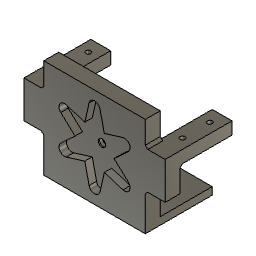
Middle_Servo_Mount (Autodesk Fusion 360 design; units mm, degrees)
Autodesk Fusion 360 part; units mm, degrees
note: some values were not read from the file. Set by a fixed rule: which sketch regions a step uses.
sketch "Sketch1" plane through (0, 0, 0) normal (0, 0, 1) x (1, 0, 0)
  line L0 (41, 21) -> (20.5, 21)
  line L1 (20.5, 21) -> (0, 21)
  line L2 (41, 0) -> (41, 21)
  line L3 (0, 21) -> (0, 0)
  line L4 (0, 0) -> (41, 0)
  dimension "d1" = 21
  dimension "d2" = 41
  constraint horizontal L4
  constraint vertical L2
  constraint horizontal L0
  constraint vertical L3
  constraint coincident L3.end L4.start
  constraint collinear L0 L1
  measures "d1" distance of L3.end L1.end
  measures "d2" distance of L3.end L2.start
extrude "Extrude1" add sketch "Sketch1" along normal blind 3
sketch "Sketch7" plane through (0, 0, 0) normal (0, 0, -1) x (1, 0, 0)
  line L0 (0, 0) -> (0, -21)
  line L1 (0, -21) -> (20.5, -21)
  line L2 (20.5, -21) -> (41, -21)
  line L3 (41, -21) -> (41, 0)
  line L4 (41, 0) -> (0, 0)
  line L5 (0, 0) -> (41, 0)
  line L6 (41, 0) -> (41, 6)
  line L7 (41, 6) -> (0, 6)
  line L8 (0, 6) -> (0, 0)
  dimension "d23" = 6
  constraint horizontal L5
  constraint vertical L6
  constraint horizontal L7
  constraint vertical L8
  measures "d23" distance of L3.end L6.end
extrude "Extrude6" add sketch "Sketch7" against normal blind 40 contours L4 L5 L6 L7 L8
sketch "Sketch8" plane through (0, -6, 0) normal (0, -1, 0) x (1, 0, 0)
  line L0 (0, 0) -> (41, 0)
  line L1 (41, 0) -> (41, 40)
  line L2 (41, 40) -> (0, 40)
  line L3 (0, 40) -> (0, 0)
  line L4 (41, 15) -> (49, 15)
  line L5 (49, 15) -> (49, 30)
  line L6 (49, 30) -> (41, 30)
  line L7 (41, 30) -> (41, 15)
  line L8 (20.5, 40) -> (20.5, 3)
  line L9 (0, 15) -> (-8, 15)
  line L10 (-8, 15) -> (-8, 30)
  line L11 (-8, 30) -> (0, 30)
  line L12 (0, 3) -> (41, 3)
  line L13 (0, 3) -> (41, 3)
  line L14 (0, 3) -> (41, 3)
  line L15 (0, 3) -> (41, 3)
  dimension "d24" = 15
  dimension "d25" = 27
  dimension "d28" = 8
  constraint horizontal L4
  constraint vertical L5
  constraint horizontal L6
  constraint vertical L7
  constraint coincident L1 L4.start
  constraint midpoint L2 L8.start
  constraint symmetric L4.start L8 L9.start
  constraint symmetric L4.end L8 L9.end
  constraint symmetric L5.end L8 L10.end
  constraint symmetric L6.end L8 L11.end
  measures "d24" distance of L4.end L5.end
  measures "d25" distance of L6 L12.end
  measures "d28" distance of L4.start L4.end
extrude "Extrude7" add sketch "Sketch8" against normal up to surface (6 mm away) contours L3 L9 L10 L11 | L1 L4 L5 L6 L7
sketch "Sketch9" plane through (0, 0, 0) normal (0, 1, 0) x (-1, 0, 0)
  line L0 (-41, 3) -> (0, 3)
  line L1 (0, 3) -> (0, 15)
  line L2 (0, 15) -> (8, 15)
  line L3 (8, 15) -> (8, 30)
  line L4 (8, 30) -> (0, 30)
  line L5 (0, 30) -> (0, 40)
  line L6 (0, 40) -> (-41, 40)
  line L7 (-41, 40) -> (-41, 30)
  line L8 (-41, 30) -> (-49, 30)
  line L9 (-49, 30) -> (-49, 15)
  line L10 (-49, 15) -> (-41, 15)
  line L11 (-41, 15) -> (-41, 3)
  line L12 (-49, 30) -> (-41, 30)
  line L13 (-41, 30) -> (-41, 25)
  line L14 (-41, 25) -> (-49, 25)
  line L15 (-49, 25) -> (-49, 30)
  line L16 (8, 30) -> (0, 30)
  line L17 (0, 30) -> (0, 25)
  line L18 (0, 25) -> (8, 25)
  line L19 (8, 25) -> (8, 30)
  dimension "d29" = 5
  dimension "d54" = 5
  constraint horizontal L12
  constraint vertical L13
  constraint horizontal L14
  constraint vertical L15
  constraint coincident L8.end L9.start
  constraint horizontal L16
  constraint vertical L17
  constraint horizontal L18
  constraint vertical L19
  constraint coincident L3.end L4.start
  measures "d29" distance of L7.end L13.end
  measures "d54" distance of L4.end L17.end
extrude "Extrude8" add sketch "Sketch9" along normal up to surface (21 mm away) contours L8 L9 L12 L13 L14 L15 | L3 L4 L16 L17 L18 L19
sketch "Sketch10" plane through (0, 0, 30) normal (0, 0, 1) x (-1, 0, 0)
  line L0 (8, -21) -> (8, 6)
  line L1 (8, 6) -> (0, 6)
  line L2 (0, 6) -> (0, 0)
  line L3 (0, 0) -> (0, -21)
  line L4 (0, -21) -> (8, -21)
  circle A0 centre (4, -16) radius 1
  circle A1 centre (4, -5) radius 1
  circle A2 centre (-45, -16) radius 1
  circle A3 centre (-45, -5) radius 1
  line L5 (-41, 0) -> (-41, -21)
  line L6 (0, 0) -> (-41, 0)
  dimension "d32" = 2
  dimension "d33" = 5
  dimension "d34" = 4
  dimension "d36" = 4
  dimension "d39" = 5
  constraint equal A0 A1
  constraint equal A0 A2
  constraint equal A0 A3
  constraint vertical A0.centre A1.centre
  constraint horizontal A0.centre A2.centre
  constraint horizontal A1.centre A3.centre
  constraint vertical A2.centre A3.centre
  measures "d32" diameter of A0
  measures "d33" distance of L4 A0.centre
  measures "d34" distance of L3 A0.centre
  measures "d36" distance of A2.centre L5
  measures "d39" distance of A1.centre L6
extrude "Extrude9" cut sketch "Sketch10" against normal blind 5 contours A0 | A1 | A2 | A3
chamfer "Chamfer1" distance 1 angle 45 2 edges at (-4, 0, 25) (45, 0, 25)
chamfer "Chamfer2" distance 1 angle 45 4 edges at (0, -3, 15) (41, -3, 15) (41, -3, 30) (0, -3, 30)
sketch "Sketch14" plane through (0, -6, 0) normal (0, -1, 0) x (1, 0, 0)
  line L0 (0, 0) -> (41, 0)
  line L1 (41, 0) -> (41, 14)
  line L2 (41, 14) -> (42, 15)
  line L3 (42, 15) -> (49, 15)
  line L4 (49, 15) -> (49, 30)
  line L5 (49, 30) -> (42, 30)
  line L6 (42, 30) -> (41, 31)
  line L7 (41, 31) -> (41, 40)
  line L8 (41, 40) -> (0, 40)
  line L9 (0, 40) -> (0, 31)
  line L10 (0, 31) -> (-1, 30)
  line L11 (-1, 30) -> (-8, 30)
  line L12 (-8, 30) -> (-8, 15)
  line L13 (-8, 15) -> (-1, 15)
  line L14 (-1, 15) -> (0, 14)
  line L15 (0, 14) -> (0, 0)
  line L16 (6.8481, 25.348) -> (12.6318, 20)
  line L17 (12.6318, 20) -> (6.8481, 14.652)
  arc A0 (6.8481, 14.652) -> (9.0425, 10.8511) centre (8.3756, 13) ccw
  line L18 (9.0425, 10.8511) -> (16.5659, 13.1859)
  line L19 (16.5659, 13.1859) -> (18.3056, 5.5031)
  arc A1 (18.3056, 5.5031) -> (22.6944, 5.5031) centre (20.5, 6) ccw
  line L20 (22.6944, 5.5031) -> (24.4341, 13.1859)
  line L21 (24.4341, 13.1859) -> (31.9575, 10.8511)
  arc A2 (31.9575, 10.8511) -> (34.1519, 14.652) centre (32.6244, 13) ccw
  line L22 (34.1519, 14.652) -> (28.3682, 20)
  line L23 (28.3682, 20) -> (34.1519, 25.348)
  arc A3 (34.1519, 25.348) -> (31.9575, 29.1489) centre (32.6244, 27) ccw
  line L24 (31.9575, 29.1489) -> (24.4341, 26.8141)
  line L25 (24.4341, 26.8141) -> (22.6944, 34.4969)
  arc A4 (22.6944, 34.4969) -> (18.3056, 34.4969) centre (20.5, 34) ccw
  line L26 (18.3056, 34.4969) -> (16.5659, 26.8141)
  line L27 (16.5659, 26.8141) -> (9.0425, 29.1489)
  arc A5 (9.0425, 29.1489) -> (6.8481, 25.348) centre (8.3756, 27) ccw
  point P0 (20.5, 20)
  dimension "d48" = 40
  dimension "d49" = 41
  measures "d48" distance of L0.start L8.end
  measures "d49" distance of L0.start L0.end
extrude "Extrude11" cut sketch "Sketch14" against normal blind 3 contours L16 L17 A0 L18 L19 A1 L20 L21 A2 L22 L23 A3 L24 L25 A4 L26 L27 A5
sketch "Sketch15" plane through (0, 0, 0) normal (0, 1, 0) x (-1, 0, 0)
  line L0 (-41, 24) -> (-49, 24)
  line L1 (-49, 24) -> (-49, 15)
  line L2 (-49, 15) -> (-42, 15)
  line L3 (-42, 15) -> (-41, 14)
  line L4 (-41, 14) -> (-41, 3)
  line L5 (-41, 3) -> (0, 3)
  line L6 (0, 3) -> (0, 14)
  line L7 (0, 14) -> (1, 15)
  line L8 (1, 15) -> (8, 15)
  line L9 (8, 15) -> (8, 24)
  line L10 (8, 24) -> (0, 24)
  line L11 (0, 24) -> (0, 30)
  line L12 (0, 30) -> (1, 30)
  line L13 (1, 30) -> (0, 31)
  line L14 (0, 31) -> (0, 40)
  line L15 (0, 40) -> (-41, 40)
  line L16 (-41, 40) -> (-41, 31)
  line L17 (-41, 31) -> (-42, 30)
  line L18 (-42, 30) -> (-41, 30)
  line L19 (-41, 30) -> (-41, 24)
  line L20 (-20.5, 40) -> (-20.5, 0)
  circle A0 centre (-20.5, 20) radius 3.25
  point P0 (-28.3682, 20)
  dimension "d53" = 6.5
  constraint midpoint L15 L20.start
  constraint perpendicular L5 L20
  constraint coincident L20 A0.centre
  constraint horizontal P0 A0.centre
  measures "d53" diameter of A0
extrude "Extrude12" cut sketch "Sketch15" against normal blind 2.5 contours L20 A0 | L20 A0
sketch "Sketch16" plane through (0, -2.5, 0) normal (0, 1, 0) x (-1, 0, 0)
  circle A0 centre (-20.5, 20) radius 3.25
  circle A1 centre (-20.5, 20) radius 1.5
  dimension "d57" = 3
  constraint coincident A0.centre A1.centre
  measures "d57" diameter of A1
extrude "Extrude13" cut sketch "Sketch16" against normal blind 0.5 contours A1
sketch "Sketch17" plane through (0, 0, 0) normal (0, 0, -1) x (1, 0, 0)
  line L0 (0, 6) -> (0, -21)
  line L1 (0, -21) -> (20.5, -21)
  line L2 (20.5, -21) -> (41, -21)
  line L3 (41, -21) -> (41, 6)
  line L4 (41, 6) -> (0, 6)
  circle A0 centre (11, -10) radius 1.5
  line L5 (0, 0) -> (41, 0)
  dimension "d60" = 30
  dimension "d61" = 10
  dimension "d62" = 3
  measures "d60" distance of L3 A0.centre
  measures "d61" distance of A0.centre L5
  measures "d62" diameter of A0
extrude "Extrude14" cut sketch "Sketch17" against normal blind 3 contours A0
sketch "Sketch18" plane through (0, 0, 3) normal (0, 0, 1) x (-1, 0, 0)
  circle A0 centre (-11, -10) radius 1.5
  line L0 (0, 0) -> (-41, 0)
  line L1 (-41, 0) -> (-41, -21)
  line L2 (-41, -21) -> (-20.5, -21)
  line L3 (-20.5, -21) -> (0, -21)
  line L4 (0, -21) -> (0, 0)
  circle A1 centre (-11, -10) radius 2.5
  dimension "d65" = 5
  dimension "d69" = 3
  constraint concentric A0 A1
  measures "d65" diameter of A1
  measures "d69" diameter of A0
extrude "Extrude15" cut sketch "Sketch18" against normal blind 2 contours A1
chamfer "Chamfer3" distance 1 angle 45 1 edges at (9.6015, 9.4576, 0)
